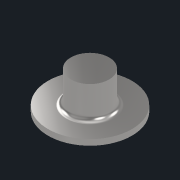
# Autodesk Inventor part: core
Saved by Autodesk Inventor 2022.2 (Build 262287010, 287A)
## iProperties
Created: 2023-07-19
Part Number: core
Material: Steel
Document SubType Name: Modeling
Designer: StijnC
Density: 7.85 g/cm^3
Appearance: Semi-Polished
Author: StijnC
Autodesk Inventor part; units mm, degrees
ref_plane "YZ Plane" through (0, 0, 0) normal (1, 0, 0) x (0, 1, 0)
ref_plane "XZ Plane" through (0, 0, 0) normal (0, 1, 0) x (-1, 0, 0)
ref_plane "XY Plane" through (0, 0, 0) normal (0, 0, 1) x (1, 0, 0)
sketch "Sketch1" plane through (0, 0, 0) normal (0, 1, 0) x (-1, 0, 0)
  circle A0 centre (0, 0) radius 8.75
  dimension "d0" = 17.5
  constraints: 1 centre point, 1 coincident
  measures "d0" diameter of A0
extrude "Extrusion1" add sketch "Sketch1" along normal blind 1.2
sketch "Sketch2" plane through (0, 1.2, 0) normal (0, 1, 0) x (1, 0, 0)
  circle A0 centre (0, 0) radius 4
  dimension "d3" = 8
  constraints: 1 centre point, 1 coincident
  measures "d3" diameter of A0
extrude "Extrusion2" add sketch "Sketch2" along normal blind 6.6
fillet "Fillet1" radius 1 1 edges at (-4, 1.2, 0)
body "Solid1"
